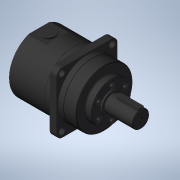
# Autodesk Inventor part: HPG-20A-11-J6GDK(400)
Saved by Autodesk Inventor 2021 (Build 250183000, 183)
## iProperties
Created: 2025-02-25
Part Number: HPG-20A-11-J6GDK(400)
Material: Generic
Catalog Web Link: www.cadenas.de
Description: HPG-20A-
Vendor: HARMONIC
Document SubType Name: Modeling
Designer: psAdmin
Manufacturer: HARMONIC
Mass: 599.167 g
Surface Area: 662.141 cm^2
Volume: 599.167 cm^3
Density: 1 g/cm^3
Appearance: PSOLRGB-175-175-175
Category: PARTsolutions
Company: HARMONIC
Title: HPG-20A-11-J6GDK
Author: Cadenas PARTsolutions
PSOL_IDENT_0: {$CADENAS_DATA/23d-libs/harmonicdrive/data/hpg_series/selection_for_order_number/3d/shaft_output_tap
PSOL_IDENT_1: ped_hole/hpg_20a_j6.prj},180 {VTYP=3D},{NB=HPG-20A-11-J6GDK(400)},{LINA=HPG-20A-11-J6GDK},{NN=HPG-20
PSOL_IDENT_2: A},{DATE=16.11.2023 08:26:27},{GEOMDATE=09.08.2021 09:58:37},{VERSION=},{LINEID=2670},{WBVAR=},{WBNU
PSOL_IDENT_3: MERIC=}  {NB=HPG-20A-11-J6GDK(400)},{LINA=HPG-20A-11-J6GDK},{KT=DUMMY},{CNSORDERNO=HPG-20A-11-J6GDK}
PSOL_IDENT_4: ,{R=11},{MC=400},{FN=GDK},{CNSORDERNO26=J6},{SB=0},{VERX=0}
NB: HPG-20A-11-J6GDK(400)
NN: HPG-20A
NBSYN: $CNSORDERNO.($MC.)
LINA: HPG-20A-11-J6GDK
CATALOG: Harmonic Drive
CNSORDERNO: HPG-20A-11-J6GDK
R: 11
MC: 400
FN: GDK
VERX: 0
SUPPLIER: HARMONIC
ARTICLENO: HPG-20A-11-J6GDK(400)
BOMINFO: HPG-20A-11-J6GDK
CREATOR: CADENAS GmbH
Autodesk Inventor part; units mm, degrees
ref_plane "YZ Plane" through (0, 0, 0) normal (1, 0, 0) x (0, 1, 0)
ref_plane "XZ Plane" through (0, 0, 0) normal (0, 1, 0) x (-1, 0, 0)
ref_plane "XY Plane" through (0, 0, 0) normal (0, 0, 1) x (1, 0, 0)
sketch "Sketch_1" plane through (0, 0, 0) normal (0, 0, 1) x (1, 0, 0)
  line L0 (151, 0) -> (35.5, 0)
  line L1 (35.5, 0) -> (35.5, 7)
  line L2 (35.5, 7) -> (9, 7)
  line L3 (9, 7) -> (9, 17.5)
  line L4 (9, 17.5) -> (24.5, 17.5)
  line L5 (24.5, 17.5) -> (24.5, 20.5)
  line L6 (24.5, 20.5) -> (27.5, 20.5)
  line L7 (27.5, 20.5) -> (27.5, 27.5)
  line L8 (27.5, 27.5) -> (10, 27.5)
  line L9 (10, 27.5) -> (10, 25)
  line L10 (10, 25) -> (0.5, 25)
  line L11 (0.5, 25) -> (0, 25.5)
  line L12 (0, 25.5) -> (0, 44)
  line L13 (0, 44) -> (0.5, 44.5)
  line L14 (0.5, 44.5) -> (52, 44.5)
  line L15 (52, 44.5) -> (52, 44)
  line L16 (52, 44) -> (52.5, 44.5)
  line L17 (52.5, 44.5) -> (71, 44.5)
  line L18 (71, 44.5) -> (71, 42.5)
  line L19 (71, 42.5) -> (78.5, 42.5)
  line L20 (78.5, 42.5) -> (79, 42)
  line L21 (79, 42) -> (96, 42)
  line L22 (96, 42) -> (97, 41)
  line L23 (97, 41) -> (97, 29.5)
  line L24 (97, 29.5) -> (97.5, 29.5)
  line L25 (97.5, 29.5) -> (98, 29)
  line L26 (98, 29) -> (98.5, 29.5)
  line L27 (98.5, 29.5) -> (106.5, 29.5)
  line L28 (106.5, 29.5) -> (107, 29)
  line L29 (107, 29) -> (107, 16)
  line L30 (107, 16) -> (109, 16)
  line L31 (109, 16) -> (109, 12.9)
  arc A0 (109, 12.9) -> (109.4, 12.5) centre (109.4, 12.9) ccw
  line L32 (109.4, 12.5) -> (150, 12.5)
  line L33 (150, 12.5) -> (151, 11.5)
  line L34 (151, 11.5) -> (151, 0)
  line L35 (151, 0) -> (35.5, 0)
  constraints: 72 end point, 2 point on circle, 1 centre point
revolve "Revolution1" add sketch "Sketch_1" angle 360 about axis through (151, 0, 0) along (1, 0, 0)
sketch "Sketch_2" plane through (0, 0, 0) normal (1, 0, 0) x (0, 1, 0)
  line L0 (61.5, 20) -> (41.5, 20)
  line L1 (41.5, 20) -> (41.5, -20)
  line L2 (41.5, -20) -> (61.5, -20)
  line L3 (61.5, -20) -> (61.5, 20)
  constraints: 8 end point
extrude "Extrusion1" cut sketch "Sketch_2" along normal blind 28
sketch "Sketch_3" plane through (0, 0, 0) normal (1, 0, 0) x (0, 1, 0)
  line L0 (0.5, 16) -> (-0.5, 16)
  line L1 (-0.5, 16) -> (-0.5, -19)
  line L2 (-0.5, -19) -> (0.5, -19)
  line L3 (0.5, -19) -> (0.5, 16)
  constraints: 8 end point
extrude "Extrusion2" cut sketch "Sketch_3" along normal blind 22
sketch "Sketch_4" plane through (14, 0, 0) normal (1, 0, 0) x (0, 0, -1)
  line L0 (13.5, -15) -> (13.5, 17)
  line L1 (13.5, 17) -> (17.5, 17)
  line L2 (17.5, 17) -> (17.5, 4)
  line L3 (17.5, 4) -> (15.75, 4)
  line L4 (15.75, 4) -> (15.75, -15)
  line L5 (15.75, -15) -> (13.5, -15)
  line L6 (13.5, -15) -> (13.5, 17)
  constraints: 14 end point
revolve "Revolution2" cut sketch "Sketch_4" angle 360 about axis through (14, -15, -13.5) along (0, -1, 0)
sketch "Sketch_5" plane through (14, 0, 0) normal (1, 0, 0) x (0, 0, -1)
  line L0 (13.5, -10) -> (13.5, 11)
  line L1 (13.5, 8) -> (16.8, 8)
  line L2 (16.8, 8) -> (17, 7.8)
  line L3 (17, 7.8) -> (17, 3)
  line L4 (17, 3) -> (15.75, 3)
  line L5 (15.75, 3) -> (15.75, -9.6)
  line L6 (15.75, -9.6) -> (15.35, -10)
  line L7 (15.35, -10) -> (13.5, -10)
  line L8 (13.5, -10) -> (13.5, 8)
  constraints: 18 end point
revolve "Revolution3" add sketch "Sketch_5" angle 360 about axis through (14, -10, -13.5) along (0, -1, 0)
sketch "Sketch_6" plane through (0, 8, 0) normal (0, 1, 0) x (1, 0, 0)
  line L0 (12.5, 12.634) -> (14, 11.7679)
  line L1 (14, 11.7679) -> (15.5, 12.634)
  line L2 (15.5, 12.634) -> (15.5, 14.366)
  line L3 (15.5, 14.366) -> (14, 15.2321)
  line L4 (14, 15.2321) -> (12.5, 14.366)
  line L5 (12.5, 14.366) -> (12.5, 12.634)
  constraints: 12 end point
extrude "Extrusion3" cut sketch "Sketch_6" against normal blind 2
sketch "Sketch_7" plane through (14, 0, 0) normal (1, 0, 0) x (0, 0, -1)
  line L0 (0, 20) -> (0, 45)
  line L1 (0, 45) -> (8.25, 45)
  line L2 (8.25, 45) -> (8.25, 20)
  line L3 (8.25, 20) -> (0, 20)
  line L4 (0, 20) -> (0, 45)
  constraints: 10 end point
revolve "Revolution4" cut sketch "Sketch_7" angle 360 about axis through (14, 20, 0) along (0, -1, 0)
sketch "Sketch_8" plane through (14, 0, 0) normal (1, 0, 0) x (0, 0, -1)
  line L0 (0, 17) -> (0, 43.5)
  line L1 (0, 43.5) -> (10, 43.5)
  arc A0 (10.5, 43) -> (10, 43.5) centre (10, 43) ccw
  line L2 (10.5, 43) -> (10.5, 41.5)
  line L3 (10.5, 41.5) -> (8, 41.5)
  line L4 (8, 41.5) -> (8, 36.5)
  line L5 (8, 36.5) -> (0, 36.5)
  line L6 (0, 36.5) -> (0, 43.5)
  constraints: 14 end point, 2 point on circle, 1 centre point
revolve "Revolution5" add sketch "Sketch_8" angle 360 about axis through (14, 17, 0) along (0, -1, 0)
sketch "Sketch_15" plane through (61, 0, 0) normal (1, 0, 0) x (0, 0, -1)
  arc A0 (-45, -36) -> (-36, -45) centre (-36, -36) ccw
  line L0 (-36, -45) -> (36, -45)
  arc A1 (36, -45) -> (45, -36) centre (36, -36) ccw
  line L1 (45, -36) -> (45, 36)
  arc A2 (45, 36) -> (36, 45) centre (36, 36) ccw
  line L2 (36, 45) -> (-36, 45)
  arc A3 (-36, 45) -> (-45, 36) centre (-36, 36) ccw
  line L3 (-45, 36) -> (-45, -36)
  circle A4 centre (37.1231, 37.1231) radius 4.5
  circle A5 centre (37.1231, -37.1231) radius 4.5
  circle A6 centre (-37.1231, 37.1231) radius 4.5
  circle A7 centre (-37.1231, -37.1231) radius 4.5
  constraints: 8 centre point, 8 end point, 8 point on circle
extrude "Extrusion4" add sketch "Sketch_15" along normal blind 10
sketch "Sketch10" plane through (0, 0, 0) normal (-1, 0, 0) x (0, 0, 1)
  point P0 (14.9247, 36.0313)
hole "Hole1" at (0, 36.0313, 14.9247) direction (1, 0, 0) diameter 8 depth 5
pattern_circular "Circular Pattern1" count 8 over 360 about axis through (0, 0, 0) along (1, 0, 0) of "Hole1"
sketch "Sketch_11" plane through (0, 0, 0) normal (0, -0.3826834, 0.9238795) x (1, 0, 0)
  line L0 (5, 39) -> (1, 39)
  line L1 (1, 39) -> (1, 42)
  line L2 (1, 42) -> (1.5, 42.5)
  line L3 (1.5, 42.5) -> (5, 42.5)
  line L4 (5, 42.5) -> (5, 39)
  line L5 (5, 39) -> (1, 39)
  constraints: 12 end point
revolve "Revolution6" add sketch "Sketch_11" angle 360 about axis through (5, 36.0313, 14.9247) along (1, 0, 0)
pattern_circular "Circular Pattern2" count 8 over 360 about axis through (1, 0, 0) along (1, 0, 0) of "Revolution6"
sketch "Sketch_13" plane through (1, 0, 0) normal (1, 0, 0) x (0, 0, -1)
  line L0 (-16.6419, 36.2574) -> (-15.9791, 34.6572)
  line L1 (-15.9791, 34.6572) -> (-14.2618, 34.4311)
  line L2 (-14.2618, 34.4311) -> (-13.2074, 35.8052)
  line L3 (-13.2074, 35.8052) -> (-13.8702, 37.4054)
  line L4 (-13.8702, 37.4054) -> (-15.5875, 37.6315)
  line L5 (-15.5875, 37.6315) -> (-16.6419, 36.2574)
  constraints: 12 end point
extrude "Extrusion5" cut sketch "Sketch_13" along normal blind 3
pattern_circular "Circular Pattern3" count 8 over 360 about axis through (1, 0, 0) along (1, 0, 0) of "Extrusion5"
sketch "Sketch13" plane through (0, 0, 0) normal (-1, 0, 0) x (0, 0, 1)
  point P0 (24.7487, 24.7487)
hole "Hole2" at (0, 24.7487, 24.7487) direction (1, 0, 0) diameter 3.242 depth 12 tip angle 120 countersink diameter 4 countersink angle 90 thread size "M4x0.7" class "6H" standard "ISO Metric profile"
pattern_linear "Rectangular Pattern1" count 2 spacing 49.4975 along (0, 0, -1) count 2 spacing 49.4975 along (0, -1, 0) of "Hole2"
sketch "Sketch14" plane through (107, 0, 0) normal (1, 0, 0) x (0, 0, -1)
  point P0 (0, 22.5)
hole "Hole3" at (107, 22.5, 0) direction (-1, 0, 0) diameter 11 depth 6
pattern_linear "Rectangular Pattern2" count 3 spacing 22.5 along (0, -0.5, 0.8660254) count 3 spacing 22.5 along (0, -0.5, -0.8660254) of "Hole3" skipped copies 3 5 7
sketch "Sketch_21" plane through (0, 0, 0) normal (0, 0, 1) x (1, 0, 0)
  line L0 (107, 22.5) -> (101, 22.5)
  line L1 (101, 22.5) -> (101, 27.5)
  line L2 (101, 27.5) -> (106.6667, 27.5)
  arc A0 (107, 27.1667) -> (106.6667, 27.5) centre (106.6667, 27.1667) ccw
  line L3 (107, 27.1667) -> (107, 22.5)
  line L4 (107, 22.5) -> (101, 22.5)
  constraints: 10 end point, 2 point on circle, 1 centre point
revolve "Revolution7" add sketch "Sketch_21" angle 360 about axis through (107, 22.5, 0) along (1, 0, 0)
pattern_linear "Rectangular Pattern3" count 3 spacing 22.5 along (0, -0.5, 0.8660254) count 3 spacing 22.5 along (0, -0.5, -0.8660254) of "Revolution7" skipped copies 3 5 7
sketch "Sketch_23" plane through (107, 0, 0) normal (1, 0, 0) x (0, 0, -1)
  line L0 (-2.5, 21.0566) -> (0, 19.6132)
  line L1 (0, 19.6132) -> (2.5, 21.0566)
  line L2 (2.5, 21.0566) -> (2.5, 23.9434)
  line L3 (2.5, 23.9434) -> (0, 25.3868)
  line L4 (0, 25.3868) -> (-2.5, 23.9434)
  line L5 (-2.5, 23.9434) -> (-2.5, 21.0566)
  constraints: 12 end point
extrude "Extrusion6" cut sketch "Sketch_23" against normal blind 3
pattern_linear "Rectangular Pattern4" count 3 spacing 22.5 along (0, -0.5, 0.8660254) count 3 spacing 22.5 along (0, -0.5, -0.8660254) of "Extrusion6" skipped copies 3 5 7
sketch "Sketch_25" plane through (0, 0, 0) normal (0, 1, 0) x (-1, 0, 0)
  line L0 (-115, -0.8) -> (-115, 0.8)
  line L1 (-115, 0.8) -> (-118.2, 4)
  line L2 (-118.2, 4) -> (-151, 4)
  line L3 (-151, 4) -> (-151, -4)
  line L4 (-151, -4) -> (-118.2, -4)
  line L5 (-118.2, -4) -> (-115, -0.8)
  constraints: 12 end point
extrude "Extrusion7" add sketch "Sketch_25" along normal blind 15.5
sketch "Sketch18" plane through (151, 10.7819, -4) normal (1, 0, 0) x (0, 0, -1)
  point P0 (-4, -10.7819)
hole "Hole4" at (151, 0, 0) direction (-1, 0, 0) diameter 4.917 depth 15 tip angle 120 countersink diameter 6 countersink angle 90 thread size "M6x1" class "6H" standard "ISO Metric profile"
sketch "Sketch_27" plane through (20, 0, 0) normal (1, 0, 0) x (0, 0, -1)
  line L0 (-5, 17.2916) -> (-5, -17.2916)
  arc A0 (-5, -17.2916) -> (-5, 17.2916) centre (0, 0) ccw
  constraints: 2 end point, 2 point on circle, 1 centre point
extrude "Extrusion8" cut sketch "Sketch_27" against normal blind 1
ref_plane "IP_XY" through (0, 0, 0) normal (1, 0, 0) x (0, 0, -1)
ref_plane "IP_YZ" through (0, 0, 0) normal (0, 0, -1) x (0, 1, 0)
ref_plane "IP_ZX" through (0, 0, 0) normal (0, 1, 0) x (1, 0, 0)
body "Solid1"
